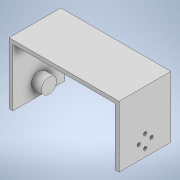
# Autodesk Inventor part: Tilt_Bracket
Saved by Autodesk Inventor 2022 (Build 260153000, 153)
## iProperties
Created: 2022-02-11
Part Number: Tilt_Bracket
Material: Generic
Document SubType Name: Modeling
Designer: Mlees
Density: 1 g/cm^3
Appearance: Default
Author: Mlees
Autodesk Inventor part; units mm, degrees
ref_plane "YZ Plane" through (0, 0, 0) normal (1, 0, 0) x (0, 1, 0)
ref_plane "XZ Plane" through (0, 0, 0) normal (0, 1, 0) x (-1, 0, 0)
ref_plane "XY Plane" through (0, 0, 0) normal (0, 0, 1) x (1, 0, 0)
sketch "Sketch1" plane through (0, 0, 0) normal (0, 0, 1) x (1, 0, 0)
  line L0 (0, 0) -> (0, 45)
  line L1 (0, 45) -> (80, 45)
  line L2 (80, 45) -> (80, 0)
  line L3 (80, 0) -> (83, 0)
  line L4 (83, 0) -> (83, 48)
  line L5 (83, 48) -> (-3, 48)
  line L6 (-3, 48) -> (-3, 0)
  line L7 (-3, 0) -> (0, 0)
  dimension "d0" = 45
  dimension "d1" = 80
  dimension "d2" = 3
  dimension "d3" = 48
  dimension "d4" = 86
  constraints: 16 end point, 6 perpendicular, 1 horizontal, 1 point on line, 1 vertical
  measures "d0" distance of L0.start L0.end
  measures "d1" distance of L0.end L1.end
  measures "d2" distance of L2.end L3.end
  measures "d3" distance of L3.end L4.end
  measures "d4" distance of L4.end L5.end
extrude "Extrusion1" add sketch "Sketch1" along normal blind 40.4
sketch "Sketch2" plane through (83, 0, 0) normal (1, 0, 0) x (0, 0, -1)
  line L0 (0, 0) -> (-40.4, 0) projected
  circle A0 centre (-20.2, 16) radius 1.25
  circle A1 centre (-25.2, 11) radius 1.25
  circle A2 centre (-20.2, 6) radius 1.25
  circle A3 centre (-15.2, 11) radius 1.25
  point P0 (-20.2, 11)
  dimension "d9" = 2.5
  dimension "d12" = 360
  constraints: 4 centre point, 9 other
  measures "d9" diameter of A0
extrude "Extrusion2" cut sketch "Sketch2" against normal up to surface (3 mm away)
sketch "Sketch3" plane through (0, 0, 0) normal (1, 0, 0) x (0, 0, -1)
  line L0 (0, 0) -> (-40.4, 0) projected
  circle A0 centre (-20.2, 11) radius 5.875
  dimension "d17" = 11.75
  constraints: 1 centre point
  measures "d17" diameter of A0
extrude "Extrusion3" add sketch "Sketch3" along normal blind 8
sketch "Sketch4" plane through (80, 0, 0) normal (-1, 0, 0) x (0, 0, 1)
  circle A0 centre (20.2, 6) radius 1.25 projected
  circle A1 centre (20.2, 16) radius 1.25 projected
  circle A2 centre (20.2, 11) radius 8
  point P0 (0, 0)
  dimension "d20" = 16
  constraints: 1 centre point
  measures "d20" diameter of A2
extrude "Extrusion4" cut sketch "Sketch4" against normal blind 1
body "Solid1"
